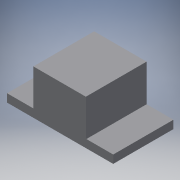
# Autodesk Inventor part: VEXButton
Saved by Autodesk Inventor 2018 (Build 220112000, 112)
## iProperties
Created: 2018-05-19
Part Number: VEXButton
Material: Generic
Document SubType Name: Modeling
Designer: reide
Density: 1 g/cm^3
Appearance: Default
Author: reide
Autodesk Inventor part; units mm, degrees
ref_plane "YZ Plane" through (0, 0, 0) normal (1, 0, 0) x (0, 1, 0)
ref_plane "XZ Plane" through (0, 0, 0) normal (0, 1, 0) x (-1, 0, 0)
ref_plane "XY Plane" through (0, 0, 0) normal (0, 0, 1) x (1, 0, 0)
sketch "Sketch1" plane through (0, 0, 0) normal (0, 0, 1) x (1, 0, 0)
  line L0 (0, 0) -> (26.55, 0)
  line L1 (26.55, 0) -> (-26.55, 0)
  line L2 (26.55, 0) -> (26.55, -15.07)
  line L3 (26.55, -15.07) -> (26.55, 15.07)
  line L4 (26.55, 15.07) -> (-26.55, 15.07)
  line L5 (-26.55, 15.07) -> (-26.55, -15.07)
  line L6 (-26.55, -15.07) -> (26.55, -15.07)
  line L7 (26.55, -15.07) -> (26.55, 15.07)
  dimension "d0" = 26.55
  dimension "d1" = 53.1
  dimension "d2" = 15.07
  dimension "d3" = 30.14
  constraints: 16 end point, 2 horizontal, 2 parallel, 2 point on line, 1 perpendicular, 1 vertical
  measures "d0" distance of L0.start L0.end
  measures "d1" distance of L0.end L1.end
  measures "d2" distance of L0.end L2.end
  measures "d3" distance of L2.end L3.end
extrude "Extrusion1" add sketch "Sketch1" along normal blind 4.05
sketch "Sketch2" plane through (0, 0, 4.05) normal (0, 0, 1) x (1, 0, 0)
  line L0 (0, 0) -> (13.125, 0)
  line L1 (13.125, 0) -> (-13.125, 0)
  line L2 (26.55, 15.07) -> (-26.55, 15.07) projected
  line L3 (13.125, 15.07) -> (-13.125, 15.07)
  line L4 (-13.125, 15.07) -> (-13.125, -15.3281)
  line L5 (13.125, -15.3281) -> (13.125, 15.07)
  line L6 (-26.55, -15.07) -> (26.55, -15.07) projected
  line L7 (13.125, 15.07) -> (-13.125, 15.07)
  line L8 (-13.125, 15.07) -> (-13.125, -15.07)
  line L9 (-13.125, -15.07) -> (13.125, -15.07)
  line L10 (13.125, -15.07) -> (13.125, 15.07)
  dimension "d6" = 13.125
  dimension "d7" = 26.25
  constraints: 18 end point, 4 point on line, 3 horizontal, 3 parallel, 2 perpendicular
  measures "d6" distance of L0.start L0.end
  measures "d7" distance of L0.end L1.end
extrude "Extrusion2" add sketch "Sketch2" along normal blind 18.45
body "Solid1"
